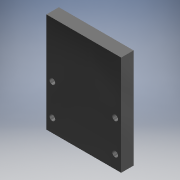
# Autodesk Inventor part: Motor spacer
Saved by Autodesk Inventor 2019 (Build 230136000, 136)
## iProperties
Part Number: Motor spacer
Material: Generic
Document SubType Name: Modeling
Designer: Delta
Appearance: Default
Author: Delta
Autodesk Inventor part; units mm, degrees
ref_plane "YZ Plane" through (0, 0, 0) normal (1, 0, 0) x (0, 1, 0)
ref_plane "XZ Plane" through (0, 0, 0) normal (0, 1, 0) x (-1, 0, 0)
ref_plane "XY Plane" through (0, 0, 0) normal (0, 0, 1) x (1, 0, 0)
sketch "Sketch1" plane through (0, 0, 0) normal (0, 0, 1) x (1, 0, 0)
  line L0 (0, 0) -> (38.1, 0)
  line L1 (38.1, 0) -> (38.1, 50.8)
  line L2 (38.1, 50.8) -> (0, 50.8)
  line L3 (0, 50.8) -> (0, 0)
  dimension "d0" = 38.1
  dimension "d1" = 50.8
  constraints: 8 end point, 2 parallel, 1 horizontal, 1 perpendicular
  measures "d0" distance of L2.end L1.end
  measures "d1" distance of L1.end L0.end
extrude "Extrusion1" add sketch "Sketch1" along normal blind 6.35
sketch "Sketch2" plane through (0, 0, 6.35) normal (0, 0, 1) x (1, 0, 0)
  line L0 (38.1, 0) -> (38.1, 50.8) projected
  line L1 (0, 0) -> (38.1, 0) projected
  circle A0 centre (35.052, 6.731) radius 1.4605
  circle A1 centre (35.052, 22.733) radius 1.4605
  dimension "d4" = 3.048
  dimension "d5" = 3.048
  dimension "d6" = 16.002
  dimension "d7" = 6.731
  dimension "d8" = 2.921
  dimension "d9" = 2.921
  constraints: 2 centre point, 2 coincident
  measures "d4" distance from line of L0 point (35.052, 6.731)
  measures "d5" distance from line of L0 point (35.052, 22.733)
  measures "d6" distance of point (35.052, 22.733) point (35.052, 6.731)
  measures "d7" distance from line of L1 point (35.052, 6.731)
  measures "d8" diameter of A0
  measures "d9" diameter of A1
extrude "Extrusion2" cut sketch "Sketch2" against normal through all
ref_plane "Work Plane1" through (19.05, 0, 0) normal (1, 0, 0) x (0, 0, -1)
mirror "Mirror1" about plane through (19.05, 0, 0) normal (1, 0, 0) of "Extrusion2"
body "Solid1"
